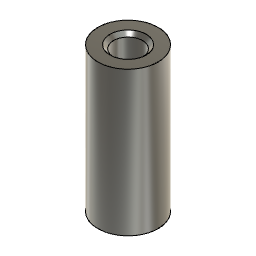
GPS-mount-extension v1 (Autodesk Fusion 360 design; units mm, degrees)
Autodesk Fusion 360 part; units mm, degrees
cylinder "CylinderPrimitive1" add diameter 5 height 12 placed x (1, 0, 0) y (0, 1, 0) z (0, 0, 1) at (0, 0, 0)
hole "Hole1" at (0.0002, 0.0066, 12) direction (0, 0, -1) diameter 2.4 depth 13 tip angle 180 countersink diameter 3 countersink angle 90
